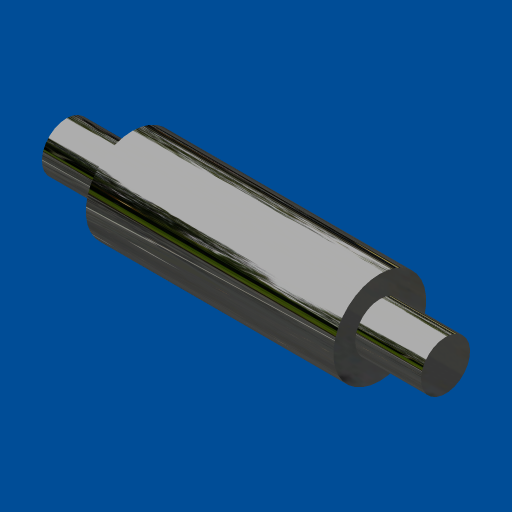
# Autodesk Inventor part: wristPin
Saved by Autodesk Inventor 2023 (Build 270158030, 158C)
## iProperties
Created: 2023-03-03
Part Number: wristPin
Material: Silicon Nitride
Document SubType Name: Modeling
Designer: kumpu
Density: 3.18 g/cm^3
Appearance: Chrome - Polished Black
Author: kumpu
Autodesk Inventor part; units mm, degrees
ref_plane "YZ Plane" through (0, 0, 0) normal (1, 0, 0) x (0, 1, 0)
ref_plane "XZ Plane" through (0, 0, 0) normal (0, 1, 0) x (-1, 0, 0)
ref_plane "XY Plane" through (0, 0, 0) normal (0, 0, 1) x (1, 0, 0)
sketch "Sketch1" plane through (0, 0, 0) normal (0, 0, 1) x (1, 0, 0)
  line L0 (-24.5, 0) -> (24.5, 0)
  line L1 (24.5, 0) -> (24.5, 3.175)
  line L2 (24.5, 3.175) -> (-24.5, 3.175)
  line L3 (-24.5, 3.175) -> (-24.5, 0)
  line L4 (-16, 3.175) -> (16, 3.175)
  line L5 (16, 3.175) -> (16, 6)
  line L6 (16, 6) -> (-16, 6)
  line L7 (-16, 6) -> (-16, 3.175)
  point P0 (0, 0)
  point P1 (0, 0)
  point P2 (0, 3.175)
  dimension "d0" = 49
  dimension "d1" = 6.35
  dimension "d2" = 32
  dimension "d3" = 12
  constraints: 16 end point, 4 parallel, 3 midpoint, 2 horizontal, 2 perpendicular, 1 coincident, 1 point on line
  measures "d0" distance of L1.end L2.end
  measures "d1" diameter of L2 L0
  measures "d2" distance of L5.end L6.end
  measures "d3" diameter of L6 L0
revolve "Revolution1" add sketch "Sketch1" angle 360 about axis through (-24.5, 0, 0) along (1, 0, 0)
body "Solid1"
